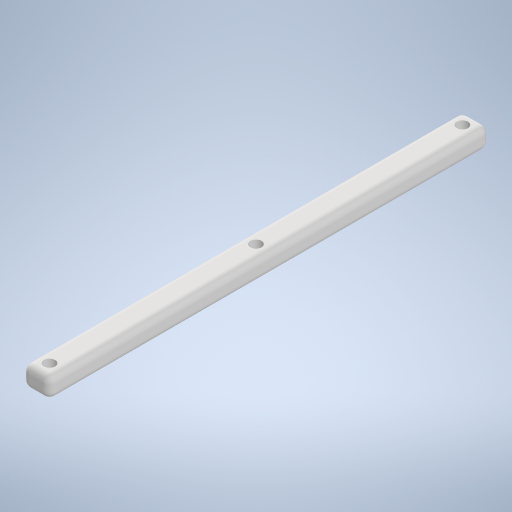
# Autodesk Inventor part: Outer bar
Saved by Autodesk Inventor 2023 (Build 270158000, 158)
## iProperties
Created: 2023-02-27
Part Number: Outer bar
Material: Generic
Document SubType Name: Modeling
Designer: Gabriel - T3 CAD
Density: 1 g/cm^3
Appearance: Default
Author: Gabriel - T3 CAD
Autodesk Inventor part; units mm, degrees
ref_plane "YZ Plane" through (0, 0, 0) normal (1, 0, 0) x (0, 1, 0)
ref_plane "XZ Plane" through (0, 0, 0) normal (0, 1, 0) x (-1, 0, 0)
ref_plane "XY Plane" through (0, 0, 0) normal (0, 0, 1) x (1, 0, 0)
sketch "Sketch1" plane through (0, 0, 0) normal (0, 1, 0) x (-1, 0, 0)
  line L0 (3.175, 0) -> (9.525, 0)
  line L1 (12.7, 3.175) -> (12.7, 200.025)
  line L2 (9.525, 203.2) -> (3.175, 203.2)
  line L3 (0, 200.025) -> (0, 3.175)
  circle A0 centre (6.35, 6.35) radius 2.5797
  circle A1 centre (6.35, 196.85) radius 2.5797
  circle A2 centre (6.35, 101.6) radius 2.5797
  arc A3 (12.7, 200.025) -> (9.525, 203.2) centre (9.525, 200.025) ccw
  arc A4 (3.175, 203.2) -> (0, 200.025) centre (3.175, 200.025) ccw
  arc A5 (0, 3.175) -> (3.175, 0) centre (3.175, 3.175) ccw
  arc A6 (9.525, 0) -> (12.7, 3.175) centre (9.525, 3.175) ccw
  point P0 (0, 0)
  point P1 (12.7, 0)
  point P2 (0, 203.2)
  dimension "d0" = 203.2
  dimension "d1" = 12.7
  dimension "d2" = 5.1594
  dimension "d3" = 6.35
  dimension "d4" = 6.35
  dimension "d5" = 5.1594
  dimension "d6" = 6.35
  dimension "d7" = 6.35
  dimension "d8" = 6.35
  dimension "d9" = 5.1594
  dimension "d10" = 101.6
  dimension "d11" = 3.175
  constraints: 8 end point, 8 point on circle, 8 tangent, 7 centre point, 6 point on line, 3 equal radius, 2 parallel, 1 horizontal, 1 perpendicular
  measures "d0" distance of point (0, 203.2) point (0, 0)
  measures "d1" distance of point (0, 0) point (12.7, 0)
  measures "d2" diameter of A0
  measures "d3" distance from line of L3 A0.centre
  measures "d4" distance from line of L0 A0.centre
  measures "d5" diameter of A1
  measures "d6" distance from line of L2 A1.centre
  measures "d7" distance from line of L3 A1.centre
  measures "d8" distance from line of L3 A2.centre
  measures "d9" diameter of A2
  measures "d10" distance from line of L0 A2.centre
  measures "d11" radius of A3
extrude "Extrusion1" add sketch "Sketch1" along normal blind 9.525
fillet "Fillet1" radius 3.175 16 edges at (-0.9299, 9.525, 0.9299) (-6.35, 9.525, 0) (-11.7701, 9.525, 0.9299) (-12.7, 9.525, 101.6) (-11.7701, 9.525, 202.2701) (-6.35, 9.525, 203.2) (-0.9299, 9.525, 202.2701) (0, 9.525, 101.6) (-0.9299, 0, 0.9299) (-6.35, 0, 0) (-11.7701, 0, 0.9299) (-12.7, 0, 101.6) (-11.7701, 0, 202.2701) (-6.35, 0, 203.2) (-0.9299, 0, 202.2701) (0, 0, 101.6)
equation "\"d3\" = 0.5 * d1"
equation "\"d4\" = d3"
equation "\"d5\" = d2"
equation "\"d6\" = d4"
equation "\"d7\" = d6"
equation "\"d8\" = d7"
equation "\"d9\" = d5"
equation "\"d10\" = 0.5 * d0"
body "Solid1"
